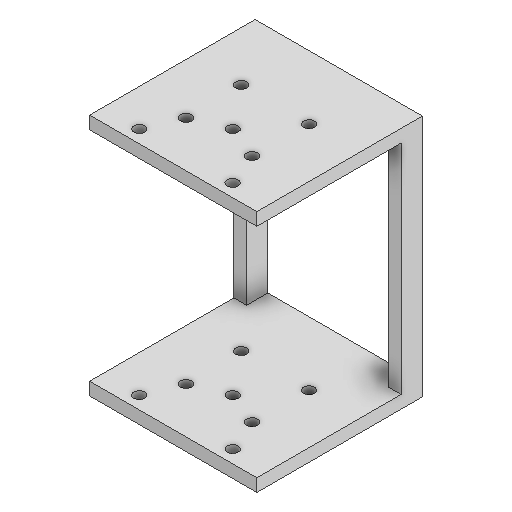
# Autodesk Inventor part: MX64 FRAME
Saved by Autodesk Inventor 2025.3 (Build 293356030, 356C)
## iProperties
Created: 2025-09-30
Part Number: MX64 FRAME
Material: 일반
Document SubType Name: Modeling
Designer: joseph
Density: 1 g/cm^3
Appearance: 기본값
Author: joseph
Autodesk Inventor part; units mm, degrees
ref_plane "YZ Plane" through (0, 0, 0) normal (1, 0, 0) x (0, 1, 0)
ref_plane "XZ Plane" through (0, 0, 0) normal (0, 1, 0) x (-1, 0, 0)
ref_plane "XY Plane" through (0, 0, 0) normal (0, 0, 1) x (1, 0, 0)
sketch "스케치1" plane through (0, 0, 0) normal (0, 0, 1) x (1, 0, 0)
  line L0 (-16.7, 25.65) -> (16.7, 25.65)
  line L1 (16.7, 25.65) -> (16.7, -25.65)
  line L2 (16.7, -25.65) -> (-16.7, -25.65)
  line L3 (-16.7, -25.65) -> (-16.7, 25.65)
  line L4 (19.7, 28.65) -> (-19.7, 28.65)
  line L5 (-19.7, 28.65) -> (-19.7, -28.65)
  line L6 (-19.7, -28.65) -> (19.7, -28.65)
  line L7 (19.7, -28.65) -> (19.7, 28.65)
  point P0 (0, 0)
  point P1 (-16.7, 0)
  point P2 (0, 25.65)
  dimension "d0" = 33.4
  dimension "d1" = 51.3
  dimension "d2" = 3
  constraints: 16 end point, 4 parallel, 2 midpoint, 2 perpendicular, 1 horizontal, 1 horizontal alignment, 1 vertical alignment, 3 other
  measures "d0" distance of L1.end L2.end
  measures "d1" distance of L0.end L1.end
  measures "d2" distance between parallel lines of L0 L4
extrude "돌출1" add sketch "스케치1" along normal blind 5
sketch "스케치5" plane through (-19.7, -28.65, 0) normal (0, -1, 0) x (1, 0, 0)
  line L0 (0, 0) -> (39.4, 0) projected
  line L1 (39.4, 0) -> (39.4, 5) projected
  line L2 (0, 5) -> (39.4, 5) projected
  line L3 (0, 0) -> (0, 5) projected
  circle A0 centre (8.7, 36) radius 1.3
  circle A1 centre (11.9218, 28.2218) radius 1.3
  circle A2 centre (19.7, 25) radius 1.3
  circle A3 centre (27.4782, 28.2218) radius 1.3
  circle A4 centre (30.7, 36) radius 1.3
  line L4 (0, 0) -> (39.4, 0)
  line L5 (39.4, 0) -> (39.4, 39)
  line L6 (39.4, 39) -> (0, 39)
  line L7 (0, 39) -> (0, 0)
  line L8 (0, 15) -> (39.4, 15) construction
  line L9 (19.7, 39) -> (19.7, 5) construction
  circle A5 centre (11.7, 15) radius 1.3
  circle A6 centre (27.7, 15) radius 1.3
  point P0 (19.7, 36)
  dimension "d46" = 180
  dimension "d52" = 39
  dimension "d53" = 24
  dimension "d54" = 2.6
  dimension "d55" = 8
  constraints: 12 end point, 7 centre point, 3 point on line, 2 midpoint, 2 parallel, 2 perpendicular, 1 horizontal, 1 symmetric about line, 10 other
  measures "d52" distance of L5.end L4.end
  measures "d53" distance between parallel lines of L6 L8
  measures "d54" diameter of A5
  measures "d55" distance from line of L9 A5.centre
extrude "돌출2" add sketch "스케치5" against normal blind 3 contours L7 L6 L5 L2
mirror "미러1" about plane through (0, 0, 0) normal (0, 1, 0)
